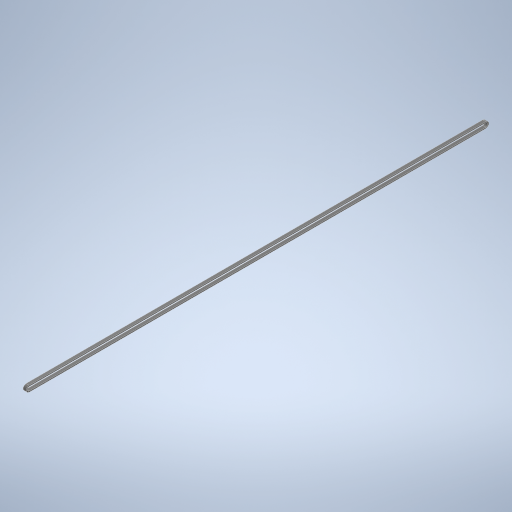
# Autodesk Inventor part: Carriage Belt
Saved by Autodesk Inventor 2023 (Build 270158000, 158)
## iProperties
Created: 2023-02-13
Part Number: Carriage Belt
Material: Generic
Document SubType Name: Modeling
Designer: mbear
Density: 1 g/cm^3
Appearance: Smooth - Black
Mass: 25.3572 g
Surface Area: 338.096 cm^2
Volume: 25.3572 cm^3
Author: mbear
Autodesk Inventor part; units mm, degrees
ref_plane "YZ Plane" through (0, 0, 0) normal (1, 0, 0) x (0, 1, 0)
ref_plane "XZ Plane" through (0, 0, 0) normal (0, 1, 0) x (-1, 0, 0)
sketch "Sketch1" plane through (0, 0, 0) normal (1, 0, 0) x (0, 1, 0)
  line L0 (3.8225, -3.8225) -> (3.8225, -892.8225)
  arc A0 (3.8225, -3.8225) -> (0, 0) centre (0, -3.8225) ccw
  arc A1 (0, 0) -> (-3.8225, -3.8225) centre (0, -3.8225) ccw
  line L1 (-3.8225, -3.8225) -> (-3.8225, -892.8225)
  arc A2 (0, -896.645) -> (3.8225, -892.8225) centre (0, -892.8225) ccw
  arc A3 (-3.8225, -892.8225) -> (0, -896.645) centre (0, -892.8225) ccw
  line L2 (0, 0) -> (0, -7.645)
  line L3 (0, -889) -> (0, -896.645)
  dimension "d0" = 896.645
  dimension "d2" = 3.8225
  dimension "d3" = 3.8225
  constraints: 12 point on circle, 8 end point, 4 centre point, 4 coincident, 3 vertical, 2 midpoint, 2 parallel, 1 concentric
  measures "d0" distance of L2.start L3.end
  measures "d2" distance of L2.start point (0, -3.822)
  measures "d3" distance of L3.end point (0, -892.822)
ref_plane "Work Plane1" through (0, 0, -3.8225) normal (0, 0, 1) x (1, 0, 0)
sketch "Sketch2" plane through (0, 0, -3.8225) normal (0, 0, 1) x (1, 0, 0)
  line L0 (-3, 5.8225) -> (3, 5.8225)
  line L1 (3, 5.8225) -> (3, 3.8225)
  line L2 (3, 3.8225) -> (-3, 3.8225)
  line L3 (-3, 3.8225) -> (-3, 5.8225)
  line L4 (0, 0) -> (0, 3.8225) projected
  point P0 (0, 0)
  point P1 (0, 5.8225)
  dimension "d5" = 2
  dimension "d6" = 0
  dimension "d7" = 6
  constraints: 8 end point, 2 parallel, 1 horizontal, 1 midpoint, 1 perpendicular, 1 vertical alignment
  measures "d5" distance between parallel lines of L2 L0
  measures "d6" distance from line of L4.end L2
  measures "d7" distance between parallel lines of L1 L3
sweep "Sweep1" add profiles "Sketch2" path "Sketch1" path curves L0 A2 A3 L1 A1 A0
body "Solid1"
